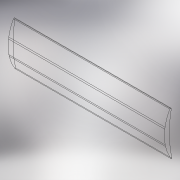
# Autodesk Inventor part: element_1
Saved by Autodesk Inventor 2018.2 (Build 222227000, 227)
## iProperties
Created: 2017-10-22
Part Number: element_1
Material: CFRP
Document SubType Name: Modeling
Designer: ku_sk
Density: 1.43 g/cm^3
Appearance: カーボンファイバー
Mass: 1502.98 g
Surface Area: 2648.54 cm^2
Volume: 1051.04 cm^3
Author: ku_sk
Autodesk Inventor part; units mm, degrees
ref_plane "YZ Plane" through (0, 0, 0) normal (1, 0, 0) x (0, 1, 0)
ref_plane "XZ Plane" through (0, 0, 0) normal (0, 1, 0) x (-1, 0, 0)
ref_plane "XY Plane" through (0, 0, 0) normal (0, 0, 1) x (1, 0, 0)
sketch "スケッチ1" plane through (0, 0, 0) normal (1, 0, 0) x (0, 1, 0)
  line L0 (0, 150) -> (0, -150)
  line L1 (-181.5936, 0) -> (756.1348, 0) projected
  arc A0 (0, 150) -> (0, -150) centre (622.1736, 0) ccw
  arc A1 (0, 150) -> (0, -150) centre (212.3676, 0) ccw
  point P0 (0, 0)
  point P1 (0, 0)
  dimension "d0" = 300
  dimension "d1" = 640
  dimension "d2" = 260
  constraints: 4 point on circle, 2 centre point, 2 end point, 2 midpoint, 1 point on line, 1 vertical
  measures "d0" distance of L0.start L0.end
  measures "d1" radius of A0
  measures "d2" radius of A1
extrude "押し出し1" add sketch "スケッチ1" along normal mid plane 950 contours A0 L1 A1 | A0 A1 L1
fillet "フィレット1" radius 5 1 edges at (0, 0, 150)
fillet "フィレット2" radius 2 1 edges at (0, 0, -150)
sketch "スケッチ2" plane through (475, 0, 0) normal (1, 0, 0) x (0, 0, -1)
  line L0 (-44.0145, -43.8798) -> (-34.1281, -45.3828)
  line L1 (59.0473, -40.8387) -> (49.2667, -42.922)
  arc A0 (-125.4594, -15.3602) -> (141.0102, -6.0726) centre (0, 212.3676) ccw projected
  point P0 (0, 0)
  dimension "d7" = 10
  dimension "d8" = 10
  constraints: 4 end point, 4 point on circle
  measures "d7" distance of L0.start L0.end
  measures "d8" distance of L1.start L1.end
extrude "押し出し2" cut sketch "スケッチ2" against normal through all
